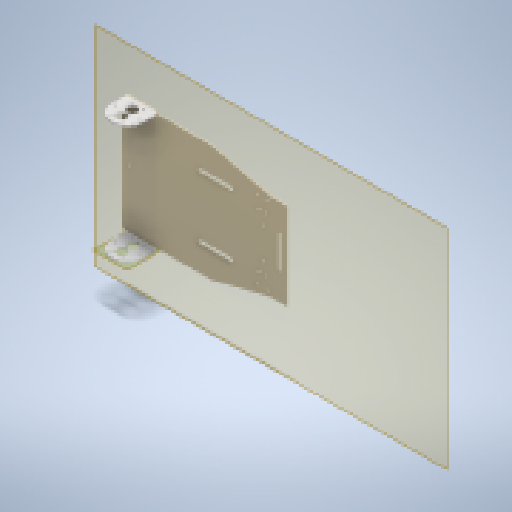
# Autodesk Inventor part: Base1
Saved by Autodesk Inventor 2023 (Build 270158000, 158)
## iProperties
Created: 2023-12-03
Part Number: Base1
Material: Genérico
Document SubType Name: Modeling
Designer: ASUS
Density: 1 g/cm^3
Appearance: Valor por defecto
Author: ASUS
Autodesk Inventor part; units mm, degrees
ref_plane "YZ Plane" through (0, 0, 0) normal (1, 0, 0) x (0, 1, 0)
ref_plane "XZ Plane" through (0, 0, 0) normal (0, 1, 0) x (-1, 0, 0)
ref_plane "XY Plane" through (0, 0, 0) normal (0, 0, 1) x (1, 0, 0)
ref_plane "Plano de trabajo1" through (0, 0, 0) normal (0, 0, 1) x (1, 0, 0)
sketch "Boceto1" plane through (0, 0, 0) normal (0, 0, 1) x (1, 0, 0)
  line L0 (14.1, -53) -> (14.1, 53)
  line L1 (-197.9, 72) -> (-197.9, -72)
  line L2 (-194.9, -75) -> (-82.9, -75)
  line L3 (-7.9, -56) -> (14.1, -56)
  line L4 (5.6, 20) -> (5.6, -20)
  line L5 (2.6, -20) -> (2.6, 20)
  circle A0 centre (4.1, -20) radius 1.5
  circle A1 centre (4.1, 20) radius 1.5
  line L6 (-14.4, 20) -> (-14.4, -20)
  line L7 (-17.4, -20) -> (-17.4, 20)
  circle A2 centre (-15.9, -20) radius 1.5
  circle A3 centre (-15.9, 20) radius 1.5
  line L8 (-12.9, -51.5) -> (-12.9, -48.5)
  line L9 (-14.4, -36.5) -> (-14.4, -33.5)
  line L10 (-21.4, -33.5) -> (-21.4, -36.5)
  line L11 (-22.9, -48.5) -> (-22.9, -51.5)
  circle A4 centre (-24.9, -50) radius 1.5
  line L12 (-22.9, -48.5) -> (-24.9, -48.5)
  line L13 (-22.9, -51.5) -> (-24.9, -51.5)
  line L14 (-10.9, -51.5) -> (-12.9, -51.5)
  line L15 (-10.9, -48.5) -> (-12.9, -48.5)
  circle A5 centre (-10.8999, -50) radius 1.5
  line L16 (-22.9, -33.5) -> (-21.4, -33.5)
  line L17 (-22.9, -36.5) -> (-21.4, -36.5)
  circle A6 centre (-22.9, -35) radius 1.5
  line L18 (-12.9, -33.5) -> (-14.4, -33.5)
  line L19 (-12.9, -36.5) -> (-14.4, -36.5)
  circle A7 centre (-12.9, -35) radius 1.5
  line L20 (-97.9, -42.5) -> (-57.9, -42.5)
  line L21 (-57.9, -37.5) -> (-97.9, -37.5)
  circle A8 centre (-57.9, -40) radius 2.5
  circle A9 centre (-97.9, -40) radius 2.5
  line L22 (14.1, 0) -> (-197.9, 0) construction
  line L23 (-12.9, 51.5) -> (-12.9, 48.5)
  line L24 (-14.4, 36.5) -> (-14.4, 33.5)
  line L25 (-21.4, 33.5) -> (-21.4, 36.5)
  line L26 (-22.9, 48.5) -> (-22.9, 51.5)
  circle A10 centre (-24.9, 50) radius 1.5
  line L27 (-22.9, 48.5) -> (-24.9, 48.5)
  line L28 (-22.9, 51.5) -> (-24.9, 51.5)
  line L29 (-10.9, 51.5) -> (-12.9, 51.5)
  line L30 (-10.9, 48.5) -> (-12.9, 48.5)
  circle A11 centre (-10.8999, 50) radius 1.5
  line L31 (-22.9, 33.5) -> (-21.4, 33.5)
  line L32 (-22.9, 36.5) -> (-21.4, 36.5)
  circle A12 centre (-22.9, 35) radius 1.5
  line L33 (-12.9, 33.5) -> (-14.4, 33.5)
  line L34 (-12.9, 36.5) -> (-14.4, 36.5)
  circle A13 centre (-12.9, 35) radius 1.5
  line L35 (-97.9, 42.5) -> (-57.9, 42.5)
  line L36 (-57.9, 37.5) -> (-97.9, 37.5)
  circle A14 centre (-57.9, 40) radius 2.5
  circle A15 centre (-97.9, 40) radius 2.5
  line L37 (-82.8999, 75) -> (-194.9, 75)
  arc A16 (-197.9, -72) -> (-194.9, -75) centre (-194.9, -72) ccw
  arc A17 (-194.9, 75) -> (-197.9, 72) centre (-194.9, 72) ccw
  arc A18 (11.1, -56) -> (14.1, -53) centre (11.1, -53) ccw
  line L38 (-7.9, 56) -> (14.1, 56)
  arc A19 (14.1, 53) -> (11.1, 56) centre (11.1, 53) ccw
  line L39 (-7.9, -56) -> (-82.9, -75)
  line L40 (-7.9, 56) -> (-82.8999, 75)
  line L41 (-197.9, 75) -> (14.1, 75)
  line L42 (14.1, 75) -> (14.1, -75)
  line L43 (14.1, -75) -> (-197.9, -75)
  line L44 (-197.9, -75) -> (-197.9, 75)
  circle A20 centre (-189.9001, 0) radius 1.5001 projected
  point P0 (0, 0)
  point P1 (14.1, 53)
  point P2 (-82.8999, 75)
  point P3 (-82.9, -75)
  point P4 (14.1, -53)
  point P5 (-97.8931, 37.5)
  point P6 (-97.8889, 42.5)
  point P7 (-57.9079, 42.5)
  point P8 (-57.9073, 37.5)
  point P9 (-22.8934, 36.5)
  point P10 (-21.4, 35.0152)
  point P11 (-21.4, 34.9847)
  point P12 (-22.8854, 33.5)
  point P13 (5.6, 19.9882)
  point P14 (5.6, -19.9951)
  point P15 (2.6, -19.9929)
  point P16 (2.6, 19.9946)
  point P17 (-21.4, -34.9847)
  point P18 (-21.4, -35.0152)
  point P19 (-22.8934, -36.5)
  point P20 (-22.8854, -33.5)
  point P21 (-97.8889, -42.5)
  point P22 (-97.8931, -37.5)
  point P23 (-57.9073, -37.5)
  point P24 (-57.9079, -42.5)
  dimension "d1" = 3
  dimension "d2" = 3
  constraints: 90 end point, 26 symmetric about line, 20 centre point, 8 point on circle, 8 tangent, 5 point on line, 2 equal radius, 2 midpoint, 2 parallel, 1 horizontal, 1 perpendicular, 6 other
  measures "d1" radius of A16
  measures "d2" radius of A19
extrude "Extrusión1" add sketch "Boceto1" against normal blind 2 contours A18 L3 L39 L2 A16 L1 A17 L37 L40 L38 A19 L0 | L42 L3 A18 | A19 L38 L42 | L6 A2 L7 A3 | L8 L15 A5 L14 | L9 A7 L19 | L9 L18 A7 | L11 L13 A4 L12 | L29 A11 L30 L23 | L34 A13 L24 | A13 L33 L24 | L27 A10 L28 L26
ref_plane "Plano de trabajo2" through (-165.025, -77.1, 12.7883) normal (0, -1, 0) x (1, 0, 0)
sketch "Boceto2" plane through (-165.025, -77.1, 12.7883) normal (0, -1, 0) x (1, 0, 0)
  line L0 (12.125, 6.7117) -> (12.125, -14.7883)
  circle A0 centre (-0.125, 20.1351) radius 1.5
  circle A1 centre (-15.6249, 20.135) radius 1.4999
  line L1 (-1.375, 13.7117) -> (-1.375, -0.2883)
  line L2 (-27.875, -14.7883) -> (-27.875, 6.7117)
  circle A2 centre (-7.8749, 13.7117) radius 6.4999
  line L3 (-14.375, -0.2883) -> (-14.375, 13.7117)
  circle A3 centre (-7.875, -0.2883) radius 6.4999
  circle A4 centre (-23.3751, 6.7116) radius 1.5001
  circle A5 centre (-15.625, -6.7117) radius 1.5
  circle A6 centre (7.625, 6.7117) radius 1.5
  line L4 (82.125, -14.7883) -> (-29.875, -14.7883)
  line L5 (-11.348, 26.4079) -> (-4.402, 26.4079)
  circle A7 centre (-0.125, -6.7117) radius 1.5
  arc A8 (12.125, 6.7117) -> (-27.875, 6.7117) centre (-7.875, 6.4055) ccw
  constraints: 12 end point, 8 centre point, 2 point on circle, 2 point on line, 2 other
extrude "Extrusión2" add sketch "Boceto2" against normal up to surface (2.1 mm away) contours L0 L4 L2 A8 | L1 A3 L3 A2
fillet "Empalme1" radius 2 1 edges at (-172.9, -77.1, -2)
mirror "Simetría1" about plane through (0, 0, 0) normal (0, 1, 0) of "Extrusión2"
